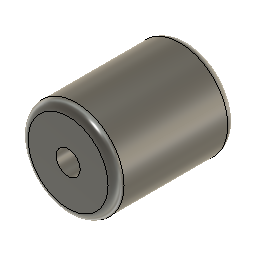
Roller Assembly (Autodesk Fusion 360 archive; units mm, degrees)
design "Roller Part"
part number: 2026-03-23-16-11-45-880
Autodesk Fusion 360 part; units mm, degrees
sketch "Sketch1" plane through (0, 0, 0) normal (0, 1, 0) x (1, 0, 0)
  circle A0 centre (0, 0) radius 15.24
  dimension "d1" = 30.48
  constraint coincident A0.centre origin
  measures "d1" diameter of A0
extrude "Extrude1" add sketch "Sketch1" along normal mid plane 38.1
fillet "Fillet1" radius 2.54 2 edges at (-14.2087, -19.05, -5.511) (-14.2087, 19.05, 5.511)
sketch "Sketch2" plane through (0, -19.05, 0) normal (0, -1, 0) x (1, 0, 0)
  circle A0 centre (0, 0) radius 12.7
  circle A1 centre (0, 0) radius 3.81
  dimension "d6" = 7.62
  constraint coincident A0.centre A1.centre
  measures "d6" diameter of A1
extrude "Extrude2" cut sketch "Sketch2" against normal through all contours A1

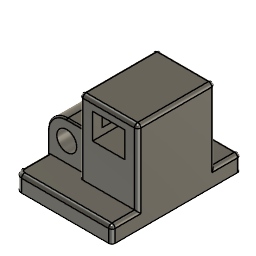
design "Front Dozer Seat"
part number: 2026-03-22-23-02-17-136
Autodesk Fusion 360 part; units mm, degrees
sketch "Sketch1" plane through (0, 0, 0) normal (0, 0, 1) x (1, 0, 0)
  line L0 (19.05, -25.4) -> (-19.05, -25.4)
  line L1 (-19.05, -25.4) -> (-19.05, 25.4)
  line L2 (-19.05, 25.4) -> (19.05, 25.4)
  line L3 (19.05, 25.4) -> (19.05, -25.4)
  line L4 (19.05, -25.4) -> (-19.05, 25.4) construction
  line L5 (-19.05, -25.4) -> (19.05, 25.4) construction
  dimension "d1" = 38.1
  dimension "d2" = 50.8
  constraint horizontal L0
  constraint perpendicular L0 L1
  constraint parallel L0 L2
  constraint parallel L1 L3
  constraint coincident L4 origin
  constraint coincident L5 origin
  measures "d1" distance of L1.end L2.end
  measures "d2" distance of L0.end L1.end
extrude "Extrude1" add sketch "Sketch1" along normal blind 6.35
sketch "Sketch2" plane through (0, 0, 6.35) normal (0, 0, 1) x (-1, 0, 0)
  line L0 (-19.05, -25.4) -> (19.05, -25.4)
  line L1 (19.05, -25.4) -> (19.05, 25.4)
  line L2 (19.05, 25.4) -> (-19.05, 25.4)
  line L3 (-19.05, 25.4) -> (-19.05, -25.4)
  line L4 (19.05, -12.7) -> (3.81, -12.7)
  line L5 (3.81, -12.7) -> (3.81, 12.7)
  line L6 (3.81, 12.7) -> (19.05, 12.7)
  line L7 (19.05, 12.7) -> (19.05, -12.7)
  line L8 (-19.05, -15.24) -> (3.81, -15.24)
  line L9 (3.81, -15.24) -> (3.81, 15.24)
  line L10 (3.81, 15.24) -> (-19.05, 15.24)
  line L11 (-19.05, 15.24) -> (-19.05, -15.24)
  dimension "d5" = 15.24
  dimension "d6" = 25.4
  dimension "d7" = 12.7
  dimension "d9" = 10.16
  dimension "d14" = 10.16
  constraint horizontal L4
  constraint vertical L5
  constraint horizontal L6
  constraint vertical L7
  constraint coincident L1 L4.start
  constraint horizontal L8
  constraint vertical L9
  constraint horizontal L10
  constraint vertical L11
  constraint coincident L3 L8.start
  constraint collinear L5 L9
  measures "d5" distance of L7 L9
  measures "d6" distance of L4 L6
  measures "d7" distance of L0 L4
  measures "d9" distance of L0 L8
  measures "d14" distance of L2 L10
extrude "Extrude2" add sketch "Sketch2" along normal blind 15.24 contours L1 L4 L5 L6 L7 L9
extrude "Extrude3" add sketch "Sketch2" along normal blind 29.21 contours L3 L5 L8 L9 L10 L11
sketch "Sketch3" plane through (0, -12.7, 0) normal (0, -1, 0) x (1, 0, 0)
  line L0 (-19.05, 6.35) -> (-3.81, 6.35)
  line L1 (-3.81, 6.35) -> (-3.81, 21.59)
  line L2 (-3.81, 21.59) -> (-19.05, 21.59)
  line L3 (-19.05, 21.59) -> (-19.05, 6.35)
  circle A0 centre (-11.43, 13.97) radius 3.937
  dimension "d15" = 7.874
  dimension "d16" = 7.62
  dimension "d17" = 7.62
  measures "d15" diameter of A0
  measures "d16" distance of L2 A0.centre
  measures "d17" distance of L3 A0.centre
extrude "Extrude4" cut sketch "Sketch3" against normal through all contours A0
fillet "Fillet1" radius 2.54 2 edges at (-19.05, -25.4, 3.175) (-19.05, 25.4, 3.175)
fillet "Fillet2" radius 1.27 6 edges at (1.27, 25.4, 6.35) (-18.3061, 24.6561, 6.35) (-19.05, 17.78, 6.35) (-19.05, -17.78, 6.35) (-18.3061, -24.6561, 6.35) (1.27, -25.4, 6.35)
fillet "Fillet3" radius 7.62 1 edges at (-19.05, 0, 21.59)
fillet "Fillet4" radius 1.27 14 edges at (-3.81, 15.24, 20.955) (7.62, 15.24, 35.56) (-3.81, 0, 35.56) (7.62, -15.24, 35.56) (-3.81, -15.24, 20.955) (19.05, 0, 35.56) (19.05, -15.24, 20.955) (19.05, 15.24, 20.955) (19.05, -25.4, 2.54) (19.05, -25.028, 5.978) (19.05, -19.685, 6.35) (19.05, 19.685, 6.35) (19.05, 25.028, 5.978) (19.05, 25.4, 2.54)
fillet "Fillet5" radius 0.508 6 edges at (-7.62, 12.7, 21.59) (-16.8182, 12.7, 19.3582) (-19.05, 12.7, 9.525) (-19.05, -12.7, 9.525) (-16.8182, -12.7, 19.3582) (-7.62, -12.7, 21.59)
sketch "Sketch4" plane through (0, 15.24, 0) normal (0, 1, 0) x (-1, 0, 0)
  line L0 (2.54, 6.35) -> (2.54, 34.29)
  line L1 (2.54, 34.29) -> (-17.78, 34.29)
  line L2 (-17.78, 34.29) -> (-17.78, 6.35)
  line L3 (-17.78, 6.35) -> (2.54, 6.35)
  line L4 (-13.97, 31.75) -> (-1.27, 31.75)
  line L5 (-1.27, 31.75) -> (-1.27, 21.59)
  line L6 (-1.27, 21.59) -> (-13.97, 21.59)
  line L7 (-13.97, 21.59) -> (-13.97, 31.75)
  dimension "d29" = 3.81
  dimension "d30" = 3.81
  dimension "d31" = 2.54
  dimension "d32" = 10.16
  constraint horizontal L4
  constraint vertical L5
  constraint horizontal L6
  constraint vertical L7
  measures "d29" distance of L2 L7
  measures "d30" distance of L0 L5
  measures "d31" distance of L1 L4
  measures "d32" distance of L4 L6
extrude "Extrude5" cut sketch "Sketch4" against normal through all contours L4 L5 L6 L7
sketch "Sketch5" plane through (-3.81, 0, 0) normal (-1, 0, 0) x (0, -1, 0)
  line L0 (13.97, 6.35) -> (13.97, 34.29)
  line L1 (13.97, 34.29) -> (-13.97, 34.29)
  line L2 (-13.97, 34.29) -> (-13.97, 6.35)
  line L3 (-13.97, 6.35) -> (-12.7, 6.35)
  line L4 (-12.7, 6.35) -> (-12.7, 21.082)
  arc A0 (-12.192, 21.59) -> (-12.7, 21.082) centre (-12.192, 21.082) ccw
  line L5 (-12.192, 21.59) -> (12.192, 21.59)
  arc A1 (12.7, 21.082) -> (12.192, 21.59) centre (12.192, 21.082) ccw
  line L6 (12.7, 21.082) -> (12.7, 6.35)
  line L7 (12.7, 6.35) -> (13.97, 6.35)
  line L8 (-11.43, 33.02) -> (11.43, 33.02)
  line L9 (11.43, 33.02) -> (11.43, 24.2438)
  line L10 (11.43, 24.2438) -> (-11.43, 24.2438)
  line L11 (-11.43, 24.2438) -> (-11.43, 33.02)
  constraint horizontal L8
  constraint vertical L9
  constraint horizontal L10
  constraint vertical L11
extrude "Extrude6" cut sketch "Sketch5" against normal up to surface (17.78 mm away) contours L8 L9 L10 L11
sketch "Sketch6" plane through (0, 0, 0) normal (0, 0, -1) x (1, 0, 0)
  arc A0 (19.05, 24.13) -> (17.78, 25.4) centre (17.78, 24.13) ccw
  line L0 (17.78, 25.4) -> (-16.51, 25.4)
  arc A1 (-16.51, 25.4) -> (-19.05, 22.86) centre (-16.51, 22.86) ccw
  line L1 (-19.05, 22.86) -> (-19.05, -22.86)
  arc A2 (-19.05, -22.86) -> (-16.51, -25.4) centre (-16.51, -22.86) ccw
  line L2 (-16.51, -25.4) -> (17.78, -25.4)
  arc A3 (17.78, -25.4) -> (19.05, -24.13) centre (17.78, -24.13) ccw
  line L3 (19.05, -24.13) -> (19.05, 24.13)
  circle A4 centre (0, 0) radius 3.5
  dimension "d36" = 7
  constraint coincident A4.centre origin
  measures "d36" diameter of A4
extrude "Extrude7" cut sketch "Sketch6" against normal blind 2 contours A4

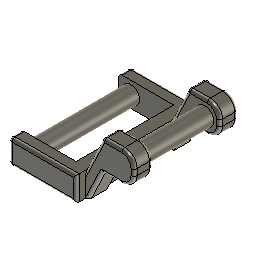
design "Roller"
part number: 2026-03-22-23-28-42-444
Autodesk Fusion 360 part; units mm, degrees
sketch "Sketch3" plane through (0, -13.97, 0) normal (0, -1, 0) x (1, 0, 0)
  line L0 (0, 10.16) -> (10.16, 10.16)
  line L1 (10.16, 10.16) -> (10.16, 20.32)
  line L2 (10.16, 20.32) -> (0, 20.32)
  line L3 (5.08, 20.32) -> (12.4091, 35.56)
  line L4 (12.4091, 35.56) -> (25.4, 35.56)
  line L5 (25.4, 35.56) -> (25.4, 22.86)
  line L6 (25.4, 22.86) -> (12.4576, 22.86)
  line L7 (12.4576, 22.86) -> (6.35, 10.16)
  line L8 (5.08, 20.32) -> (0, 20.32)
  line L9 (0, 10.16) -> (6.35, 10.16)
  line L10 (0, 20.32) -> (0, 10.16)
  line L11 (-25.4, 0) -> (0, 0)
  line L12 (0, 20.32) -> (0, 10.16)
  dimension "d22" = 25.4
  dimension "d23" = 22.86
  dimension "d24" = 12.7
  constraint perpendicular L4 L5
  constraint perpendicular L5 L6
  constraint parallel L3 L7
  constraint midpoint L2 L3.start
  constraint coincident L2.end L8.end
  constraint coincident L0.start L9.start
  measures "d22" distance of L5 L10
  measures "d23" distance of L6 L11
  measures "d24" distance of L4 L6
extrude "Extrude3" add sketch "Sketch3" along normal blind 7.62 contours L0 L1 L2 L7 L8 L9 L10 L12 | L1 L2 L3 L4 L5 L6 L7 makes body 1
mirror "Mirror1" about plane through (0, 0, 0) normal (0, 1, 0) of "Extrude3" makes body 2
sketch "Sketch4" plane through (0, -13.97, 0) normal (0, 1, 0) x (-1, 0, 0)
  line L0 (0, 20.32) -> (-5.08, 20.32)
  line L1 (-5.08, 20.32) -> (-12.4091, 35.56)
  line L2 (-12.4091, 35.56) -> (-25.4, 35.56)
  line L3 (-25.4, 35.56) -> (-25.4, 22.86)
  line L4 (-25.4, 22.86) -> (-12.4576, 22.86)
  line L5 (-12.4576, 22.86) -> (-6.35, 10.16)
  circle A0 centre (-19.346, 29.21) radius 3.683
  line L6 (-32.4673, 29.21) -> (-5.1482, 29.21) construction
  line L7 (-6.35, 10.16) -> (0, 10.16)
  line L8 (0, 10.16) -> (0, 20.32)
  dimension "d19" = 7.366
  constraint perpendicular L3 L6
  constraint coincident A0.centre L6
  measures "d19" diameter of A0
extrude "Extrude4" add sketch "Sketch4" along normal up to surface (27.94 mm away) contours A0 bodies 1
sketch "Sketch9" plane through (0, -21.59, 0) normal (0, -1, 0) x (1, 0, 0)
  line L0 (6.35, 10.16) -> (12.4576, 22.86)
  line L1 (12.4576, 22.86) -> (25.4, 22.86)
  line L2 (25.4, 22.86) -> (25.4, 35.56)
  line L3 (25.4, 35.56) -> (12.4091, 35.56)
  line L4 (12.4091, 35.56) -> (5.08, 20.32)
  line L5 (5.08, 20.32) -> (0, 20.32)
  line L6 (0, 20.32) -> (0, 10.16)
  line L7 (0, 10.16) -> (6.35, 10.16)
  line L8 (0, 20.32) -> (5.08, 20.32)
  line L9 (5.08, 20.32) -> (5.08, 10.16)
  line L10 (5.08, 10.16) -> (0, 10.16)
  line L11 (0, 10.16) -> (0, 20.32)
  dimension "d57" = 5.08
  constraint horizontal L8
  constraint vertical L9
  constraint horizontal L10
  constraint vertical L11
  constraint coincident L7 L9.end
  constraint coincident L5.end L6.start
  measures "d57" distance of L9 L11
extrude "Extrude10" add sketch "Sketch9" along normal blind 3.81 contours L5 L6 L7 L8 L9 L10 L11 bodies 1
sketch "Sketch10" plane through (0, 21.59, 0) normal (0, 1, 0) x (-1, 0, 0)
  line L0 (-12.4576, 22.86) -> (-6.35, 10.16)
  line L1 (-6.35, 10.16) -> (0, 10.16)
  line L2 (0, 10.16) -> (0, 20.32)
  line L3 (0, 20.32) -> (-5.08, 20.32)
  line L4 (-5.08, 20.32) -> (-12.4091, 35.56)
  line L5 (-12.4091, 35.56) -> (-25.4, 35.56)
  line L6 (-25.4, 35.56) -> (-25.4, 22.86)
  line L7 (-25.4, 22.86) -> (-12.4576, 22.86)
  line L8 (0, 20.32) -> (-5.08, 20.32)
  line L9 (-5.08, 20.32) -> (-5.08, 10.16)
  line L10 (-5.08, 10.16) -> (0, 10.16)
  line L11 (0, 10.16) -> (0, 20.32)
  dimension "d54" = 5.08
  constraint horizontal L8
  constraint vertical L9
  constraint horizontal L10
  constraint vertical L11
  constraint coincident L1 L9.end
  constraint coincident L2.end L3.start
  measures "d54" distance of L9 L11
extrude "Extrude11" add sketch "Sketch10" along normal blind 3.81 contours L1 L2 L3 L8 L9 L10 L11 bodies 2
sketch "Sketch11" plane through (0, 0, 0) normal (-1, 0, 0) x (0, -1, 0)
  line L0 (-13.97, 10.16) -> (-13.97, 20.32)
  line L1 (-13.97, 20.32) -> (-25.4, 20.32)
  line L2 (-25.4, 20.32) -> (-25.4, 10.16)
  line L3 (-25.4, 10.16) -> (-13.97, 10.16)
  line L4 (-25.4, 20.32) -> (-20.32, 20.32)
  line L5 (-20.32, 20.32) -> (-20.32, 10.16)
  line L6 (-20.32, 10.16) -> (-25.4, 10.16)
  line L7 (-25.4, 10.16) -> (-25.4, 20.32)
  line L8 (25.4, 20.32) -> (20.32, 20.32)
  line L9 (20.32, 20.32) -> (20.32, 10.16)
  line L10 (20.32, 10.16) -> (25.4, 10.16)
  line L11 (25.4, 10.16) -> (25.4, 20.32)
  line L12 (25.4, 20.32) -> (25.4, 10.16)
  line L13 (13.97, 20.32) -> (25.4, 20.32)
  dimension "d58" = 5.08
  dimension "d59" = 10.16
  dimension "d60" = 5.08
  dimension "d61" = 10.16
  constraint horizontal L4
  constraint vertical L5
  constraint horizontal L6
  constraint vertical L7
  constraint coincident L1.end L2.start
  constraint horizontal L8
  constraint vertical L9
  constraint horizontal L10
  constraint vertical L11
  constraint collinear L11 L12
  constraint collinear L8 L13
  measures "d58" distance of L1.end L4.end
  measures "d59" distance of L1.end L2.end
  measures "d60" distance of L8.start L8.end
  measures "d61" distance of L8.start L10.end
extrude "Extrude12" add sketch "Sketch11" along normal blind 22.86 contours L1 L2 L3 L4 L5 L6 L7 | L8 L9 L10 L11 L12 L13 bodies 1 2
sketch "Sketch12" plane through (0, 20.32, 0) normal (0, -1, 0) x (1, 0, 0)
  line L0 (0, 10.16) -> (0, 20.32)
  line L1 (0, 20.32) -> (-22.86, 20.32)
  line L2 (-22.86, 20.32) -> (-22.86, 10.16)
  line L3 (-22.86, 10.16) -> (0, 10.16)
  circle A0 centre (-17.78, 15.24) radius 3.556
  dimension "d64" = 7.112
  dimension "d65" = 5.08
  dimension "d66" = 5.08
  measures "d64" diameter of A0
  measures "d65" distance of L2 A0.centre
  measures "d66" distance of L3 A0.centre
extrude "Extrude13" add sketch "Sketch12" along normal up to surface (40.64 mm away) contours A0 bodies 1 2
sketch "Sketch13" plane through (0, 13.97, 0) normal (0, -1, 0) x (1, 0, 0)
  line L0 (6.35, 10.16) -> (12.4576, 22.86)
  line L1 (12.4576, 22.86) -> (25.4, 22.86)
  line L2 (25.4, 22.86) -> (25.4, 35.56)
  line L3 (25.4, 35.56) -> (12.4091, 35.56)
  line L4 (12.4091, 35.56) -> (5.08, 20.32)
  line L5 (5.08, 20.32) -> (0, 20.32)
  line L6 (0, 20.32) -> (0, 10.16)
  line L7 (0, 10.16) -> (6.35, 10.16)
  circle A0 centre (19.346, 29.21) radius 3.683
  line L8 (5.08, 20.32) -> (0, 20.32)
  line L9 (0, 20.32) -> (0, 10.16)
  line L10 (0, 10.16) -> (5.08, 10.16)
  line L11 (5.08, 10.16) -> (5.08, 20.32)
  constraint horizontal L8
  constraint vertical L9
  constraint horizontal L10
  constraint vertical L11
  constraint coincident L6.end L7.start
  constraint coincident L4.end L5.start
extrude "Extrude14" add sketch "Sketch13" along normal up to surface (27.94 mm away) contours L5 L6 L7 L8 L9 L10 L11 bodies 1
fillet "Fillet5" radius 5.08 4 edges at (25.4, 17.78, 35.56) (25.4, 17.78, 22.86) (25.4, -17.78, 35.56) (25.4, -17.78, 22.86) on bodies 1
fillet "Fillet6" radius 1.27 6 edges at (-22.86, -22.86, 20.32) (-22.86, -25.4, 15.24) (-8.89, -25.4, 20.32) (-22.86, -22.86, 10.16) (-8.89, -25.4, 10.16) (5.08, -25.4, 15.24) on bodies 1
fillet "Fillet7" radius 1.27 1 faces at (-4.2333, 25.4, 13.5467) on bodies 1
fillet "Fillet8" radius 1.27 4 edges at (-22.86, 22.225, 20.32) (-22.488, 25.028, 19.948) (-22.488, 25.028, 10.532) (-22.86, 22.225, 10.16) on bodies 1
fillet "Fillet9" radius 1.27 24 edges at (9.4038, -21.59, 16.51) (8.7446, -21.59, 27.94) (16.3888, -21.59, 22.86) (23.9121, -21.59, 24.3479) (25.4, -21.59, 29.21) (23.9121, -21.59, 34.0721) (16.3646, -21.59, 35.56) (16.3888, -13.97, 22.86) (23.9121, -13.97, 24.3479) (25.4, -13.97, 29.21) (23.9121, -13.97, 34.0721) (16.3646, -13.97, 35.56) (16.3646, 13.97, 35.56) (23.9121, 13.97, 34.0721) (25.4, 13.97, 29.21) (23.9121, 13.97, 24.3479) (16.3888, 13.97, 22.86) (16.3888, 21.59, 22.86) (23.9121, 21.59, 24.3479) (25.4, 21.59, 29.21) (23.9121, 21.59, 34.0721) (16.3646, 21.59, 35.56) (9.4038, 21.59, 16.51) (8.7446, 21.59, 27.94) on bodies 1
fillet "Fillet10" radius 1.27 8 edges at (8.4392, 13.97, 27.305) (12.2303, 14.342, 35.188) (12.4091, 17.78, 35.56) (12.643, 21.218, 35.188) (8.4392, -13.97, 27.305) (12.2303, -14.342, 35.188) (12.4091, -17.78, 35.56) (12.643, -21.218, 35.188) on bodies 1
fillet "Fillet11" radius 0.254 7 edges at (5.715, -13.97, 10.16) (5.08, 0, 10.16) (5.715, 13.97, 10.16) (6.35, 17.145, 10.16) (5.9853, 21.1725, 10.16) (6.35, -17.145, 10.16) (5.9853, -21.1725, 10.16) on bodies 1
